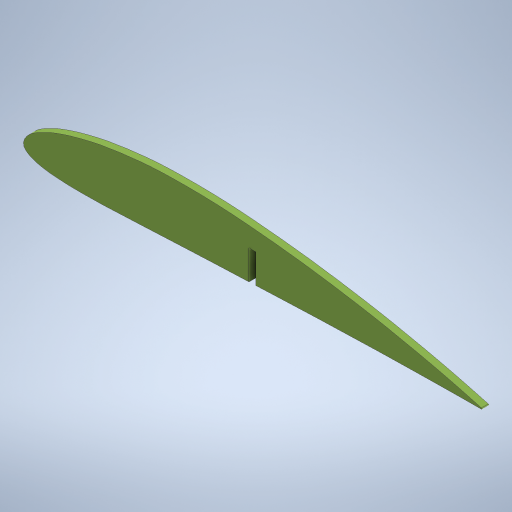
# Autodesk Inventor part: 4412_v1
Saved by Autodesk Inventor 2023 (Build 270158000, 158)
## iProperties
Created: 2023-03-24
Part Number: 4412_v1
Material: 一般
Document SubType Name: Modeling
Designer: USER
Density: 1 g/cm^3
Appearance: 預設
Author: USER
Autodesk Inventor part; units mm, degrees
ref_plane "YZ Plane" through (0, 0, 0) normal (1, 0, 0) x (0, 1, 0)
ref_plane "XZ Plane" through (0, 0, 0) normal (0, 1, 0) x (-1, 0, 0)
ref_plane "XY Plane" through (0, 0, 0) normal (0, 0, 1) x (1, 0, 0)
sketch "草圖1" plane through (0, 0, 0) normal (0, 0, 1) x (1, 0, 0)
  line L0 (0, 0) -> (200, 0)
  spline S0 degree 5 poles (200, 0.26) (199.5446, 0.3844) (198.643, 0.6302) (197.3181, 0.9903) (195.6063, 1.453) (193.5543, 2.0031) (191.5787, 2.5275) (189.6569, 3.0313) (187.7508, 3.5231) (185.8051, 4.0154) (183.7585, 4.5216) (181.5544, 5.0544) (179.1503, 5.6225) (176.5302, 6.2285) (173.7086, 6.8677) (170.7206, 7.5304) (167.6153, 8.2039) (164.4478, 8.8744) (161.2711, 9.5287) (158.1294, 10.1562) (155.049, 10.7515) (152.0374, 11.3137) (149.089, 11.8454) (146.1883, 12.3515) (143.3146, 12.838) (140.4456, 13.3106) (137.5617, 13.7738) (134.6503, 14.2291) (131.7054, 14.6761) (128.7263, 15.1128) (125.7172, 15.536) (122.6855, 15.9427) (119.6411, 16.3299) (116.5958, 16.6958) (113.5615, 17.0403) (110.5493, 17.3644) (107.5679, 17.6696) (104.622, 17.9576) (101.7109, 18.2296) (98.8272, 18.4862) (95.9547, 18.7266) (93.0695, 18.9482) (90.1456, 19.148) (87.1597, 19.3223) (84.0961, 19.4676) (80.9521, 19.5813) (77.742, 19.6616) (74.5041, 19.7086) (71.2944, 19.7241) (68.1764, 19.7106) (65.2112, 19.671) (62.448, 19.6081) (59.9142, 19.524) (57.6056, 19.4194) (55.4772, 19.2935) (53.4603, 19.1445) (51.4808, 18.9706) (49.475, 18.7707) (47.4102, 18.5458) (45.2937, 18.2988) (43.1539, 18.033) (41.0254, 17.7504) (38.934, 17.4502) (36.8779, 17.1267) (34.8276, 16.7703) (32.7467, 16.3712) (30.607, 15.9227) (28.4044, 15.4243) (26.179, 14.8861) (24.0032, 14.3258) (21.9558, 13.764) (20.1015, 13.2199) (18.469, 12.7066) (17.0265, 12.2268) (15.7021, 11.7703) (14.4082, 11.3134) (13.0653, 10.8144) (11.6221, 10.2236) (10.0713, 9.5131) (8.4648, 8.6999) (6.934, 7.8762) (5.6123, 7.1405) (4.5725, 6.5405) (3.7219, 5.9828) (2.8346, 5.2495) (1.7625, 4.1589) (0.6692, 2.7324) (-0.0769, 1.1595) (-0.1407, -0.3236) (0.5512, -1.5343) (1.6727, -2.4287) (2.8099, -3.0466) (3.7582, -3.4781) (4.6879, -3.8221) (5.8475, -4.1567) (7.301, -4.4987) (8.9432, -4.8213) (10.6131, -5.0854) (12.187, -5.2714) (13.6369, -5.3945) (14.9928, -5.4819) (16.3281, -5.5594) (17.7357, -5.6344) (19.3032, -5.7026) (21.0893, -5.7553) (23.0929, -5.7872) (25.2592, -5.798) (27.5089, -5.79) (29.7601, -5.7666) (31.9526, -5.7308) (34.0742, -5.6837) (36.1467, -5.625) (38.2074, -5.5539) (40.2921, -5.4701) (42.4166, -5.375) (44.563, -5.2721) (46.698, -5.1658) (48.7889, -5.0604) (50.8183, -4.9588) (52.8042, -4.8613) (54.8025, -4.7653) (56.8859, -4.6667) (59.127, -4.5612) (61.5817, -4.4455) (64.2685, -4.3186) (67.1689, -4.1818) (70.2406, -4.0382) (73.4254, -3.8914) (76.6596, -3.7455) (79.8838, -3.6039) (83.0524, -3.4692) (86.1437, -3.3421) (89.1553, -3.2219) (92.0991, -3.1068) (94.9966, -2.9948) (97.8733, -2.8834) (100.7544, -2.7707) (103.6595, -2.6554) (106.5987, -2.5371) (109.5748, -2.4164) (112.585, -2.2942) (115.6219, -2.1719) (118.6749, -2.0509) (121.7322, -1.9326) (124.7818, -1.8179) (127.8126, -1.7074) (130.816, -1.6015) (133.7865, -1.5002) (136.7231, -1.4033) (139.6303, -1.3107) (142.5187, -1.2221) (145.4072, -1.1373) (148.3186, -1.0562) (151.2753, -0.9786) (154.2954, -0.9047) (157.3876, -0.8343) (160.5477, -0.7676) (163.7537, -0.7048) (166.9627, -0.6461) (170.1209, -0.5918) (173.1707, -0.5421) (176.0595, -0.4974) (178.7477, -0.4575) (181.2159, -0.4226) (183.4759, -0.3922) (185.569, -0.3661) (187.5529, -0.3435) (189.4913, -0.324) (191.4427, -0.3071) (193.4484, -0.2923) (195.5324, -0.2795) (197.2722, -0.2708) (198.6195, -0.2651) (199.5367, -0.2616) (200, -0.26) knots 0 0 0 0 0 0 0.005882 0.011765 0.017647 0.023529 0.029412 0.035294 0.041176 0.047059 0.052941 0.058824 0.064706 0.070588 0.076471 0.082353 0.088235 0.094118 0.1 0.105882 0.111765 0.117647 0.123529 0.129412 0.135294 0.141176 0.147059 0.152941 0.158824 0.164706 0.170588 0.176471 0.182353 0.188235 0.194118 0.2 0.205882 0.211765 0.217647 0.223529 0.229412 0.235294 0.241176 0.247059 0.252941 0.258824 0.264706 0.270588 0.276471 0.282353 0.288235 0.294118 0.3 0.305882 0.311765 0.317647 0.323529 0.329412 0.335294 0.341176 0.347059 0.352941 0.358824 0.364706 0.370588 0.376471 0.382353 0.388235 0.394118 0.4 0.405882 0.411765 0.417647 0.423529 0.429412 0.435294 0.441176 0.447059 0.452941 0.458824 0.464706 0.470588 0.476471 0.482353 0.488235 0.494118 0.5 0.505882 0.511765 0.517647 0.523529 0.529412 0.535294 0.541176 0.547059 0.552941 0.558824 0.564706 0.570588 0.576471 0.582353 0.588235 0.594118 0.6 0.605882 0.611765 0.617647 0.623529 0.629412 0.635294 0.641176 0.647059 0.652941 0.658824 0.664706 0.670588 0.676471 0.682353 0.688235 0.694118 0.7 0.705882 0.711765 0.717647 0.723529 0.729412 0.735294 0.741176 0.747059 0.752941 0.758824 0.764706 0.770588 0.776471 0.782353 0.788235 0.794118 0.8 0.805882 0.811765 0.817647 0.823529 0.829412 0.835294 0.841176 0.847059 0.852941 0.858824 0.864706 0.870588 0.876471 0.882353 0.888235 0.894118 0.9 0.905882 0.911765 0.917647 0.923529 0.929412 0.935294 0.941176 0.947059 0.952941 0.958824 0.964706 0.970588 0.976471 0.982353 0.988235 0.994118 1 1 1 1 1 1 weights 1 1 1 1 1 1 1 1 1 1 1 1 1 1 1 1 1 1 1 1 1 1 1 1 1 1 1 1 1 1 1 1 1 1 1 1 1 1 1 1 1 1 1 1 1 1 1 1 1 1 1 1 1 1 1 1 1 1 1 1 1 1 1 1 1 1 1 1 1 1 1 1 1 1 1 1 1 1 1 1 1 1 1 1 1 1 1 1 1 1 1 1 1 1 1 1 1 1 1 1 1 1 1 1 1 1 1 1 1 1 1 1 1 1 1 1 1 1 1 1 1 1 1 1 1 1 1 1 1 1 1 1 1 1 1 1 1 1 1 1 1 1 1 1 1 1 1 1 1 1 1 1 1 1 1 1 1 1 1 1 1 1 1 1 1 1 1 1 1 1 1 1 1 1 1
  line L1 (200, 0.26) -> (199.5446, 0.3844) construction
  line L2 (199.5446, 0.3844) -> (198.643, 0.6302) construction
  line L3 (198.643, 0.6302) -> (197.3181, 0.9903) construction
  line L4 (197.3181, 0.9903) -> (195.6063, 1.453) construction
  line L5 (195.6063, 1.453) -> (193.5543, 2.0031) construction
  line L6 (193.5543, 2.0031) -> (191.5787, 2.5275) construction
  line L7 (191.5787, 2.5275) -> (189.6569, 3.0313) construction
  line L8 (189.6569, 3.0313) -> (187.7508, 3.5231) construction
  line L9 (187.7508, 3.5231) -> (185.8051, 4.0154) construction
  line L10 (185.8051, 4.0154) -> (183.7585, 4.5216) construction
  line L11 (183.7585, 4.5216) -> (181.5544, 5.0544) construction
  line L12 (181.5544, 5.0544) -> (179.1503, 5.6225) construction
  line L13 (179.1503, 5.6225) -> (176.5302, 6.2285) construction
  line L14 (176.5302, 6.2285) -> (173.7086, 6.8677) construction
  line L15 (173.7086, 6.8677) -> (170.7206, 7.5304) construction
  line L16 (170.7206, 7.5304) -> (167.6153, 8.2039) construction
  line L17 (167.6153, 8.2039) -> (164.4478, 8.8744) construction
  line L18 (164.4478, 8.8744) -> (161.2711, 9.5287) construction
  line L19 (161.2711, 9.5287) -> (158.1294, 10.1562) construction
  line L20 (158.1294, 10.1562) -> (155.049, 10.7515) construction
  line L21 (155.049, 10.7515) -> (152.0374, 11.3137) construction
  line L22 (152.0374, 11.3137) -> (149.089, 11.8454) construction
  line L23 (149.089, 11.8454) -> (146.1883, 12.3515) construction
  line L24 (146.1883, 12.3515) -> (143.3146, 12.838) construction
  line L25 (143.3146, 12.838) -> (140.4456, 13.3106) construction
  line L26 (140.4456, 13.3106) -> (137.5617, 13.7738) construction
  line L27 (137.5617, 13.7738) -> (134.6503, 14.2291) construction
  line L28 (134.6503, 14.2291) -> (131.7054, 14.6761) construction
  line L29 (131.7054, 14.6761) -> (128.7263, 15.1128) construction
  line L30 (128.7263, 15.1128) -> (125.7172, 15.536) construction
  line L31 (125.7172, 15.536) -> (122.6855, 15.9427) construction
  line L32 (122.6855, 15.9427) -> (119.6411, 16.3299) construction
  line L33 (119.6411, 16.3299) -> (116.5958, 16.6958) construction
  line L34 (116.5958, 16.6958) -> (113.5615, 17.0403) construction
  line L35 (113.5615, 17.0403) -> (110.5493, 17.3644) construction
  line L36 (110.5493, 17.3644) -> (107.5679, 17.6696) construction
  line L37 (107.5679, 17.6696) -> (104.622, 17.9576) construction
  line L38 (104.622, 17.9576) -> (101.7109, 18.2296) construction
  line L39 (101.7109, 18.2296) -> (98.8272, 18.4862) construction
  line L40 (98.8272, 18.4862) -> (95.9547, 18.7266) construction
  line L41 (95.9547, 18.7266) -> (93.0695, 18.9482) construction
  line L42 (93.0695, 18.9482) -> (90.1456, 19.148) construction
  line L43 (90.1456, 19.148) -> (87.1597, 19.3223) construction
  line L44 (87.1597, 19.3223) -> (84.0961, 19.4676) construction
  line L45 (84.0961, 19.4676) -> (80.9521, 19.5813) construction
  line L46 (80.9521, 19.5813) -> (77.742, 19.6616) construction
  line L47 (77.742, 19.6616) -> (74.5041, 19.7086) construction
  line L48 (74.5041, 19.7086) -> (71.2944, 19.7241) construction
  line L49 (71.2944, 19.7241) -> (68.1764, 19.7106) construction
  line L50 (68.1764, 19.7106) -> (65.2112, 19.671) construction
  line L51 (65.2112, 19.671) -> (62.448, 19.6081) construction
  line L52 (62.448, 19.6081) -> (59.9142, 19.524) construction
  line L53 (59.9142, 19.524) -> (57.6056, 19.4194) construction
  line L54 (57.6056, 19.4194) -> (55.4772, 19.2935) construction
  line L55 (55.4772, 19.2935) -> (53.4603, 19.1445) construction
  line L56 (53.4603, 19.1445) -> (51.4808, 18.9706) construction
  line L57 (51.4808, 18.9706) -> (49.475, 18.7707) construction
  line L58 (49.475, 18.7707) -> (47.4102, 18.5458) construction
  line L59 (47.4102, 18.5458) -> (45.2937, 18.2988) construction
  line L60 (45.2937, 18.2988) -> (43.1539, 18.033) construction
  line L61 (43.1539, 18.033) -> (41.0254, 17.7504) construction
  line L62 (41.0254, 17.7504) -> (38.934, 17.4502) construction
  line L63 (38.934, 17.4502) -> (36.8779, 17.1267) construction
  line L64 (36.8779, 17.1267) -> (34.8276, 16.7703) construction
  line L65 (34.8276, 16.7703) -> (32.7467, 16.3712) construction
  line L66 (32.7467, 16.3712) -> (30.607, 15.9227) construction
  line L67 (30.607, 15.9227) -> (28.4044, 15.4243) construction
  line L68 (28.4044, 15.4243) -> (26.179, 14.8861) construction
  line L69 (26.179, 14.8861) -> (24.0032, 14.3258) construction
  line L70 (24.0032, 14.3258) -> (21.9558, 13.764) construction
  line L71 (21.9558, 13.764) -> (20.1015, 13.2199) construction
  line L72 (20.1015, 13.2199) -> (18.469, 12.7066) construction
  line L73 (18.469, 12.7066) -> (17.0265, 12.2268) construction
  line L74 (17.0265, 12.2268) -> (15.7021, 11.7703) construction
  line L75 (15.7021, 11.7703) -> (14.4082, 11.3134) construction
  line L76 (14.4082, 11.3134) -> (13.0653, 10.8144) construction
  line L77 (13.0653, 10.8144) -> (11.6221, 10.2236) construction
  line L78 (11.6221, 10.2236) -> (10.0713, 9.5131) construction
  line L79 (10.0713, 9.5131) -> (8.4648, 8.6999) construction
  line L80 (8.4648, 8.6999) -> (6.934, 7.8762) construction
  line L81 (6.934, 7.8762) -> (5.6123, 7.1405) construction
  line L82 (5.6123, 7.1405) -> (4.5725, 6.5405) construction
  line L83 (4.5725, 6.5405) -> (3.7219, 5.9828) construction
  line L84 (3.7219, 5.9828) -> (2.8346, 5.2495) construction
  line L85 (2.8346, 5.2495) -> (1.7625, 4.1589) construction
  line L86 (1.7625, 4.1589) -> (0.6692, 2.7324) construction
  line L87 (0.6692, 2.7324) -> (-0.0769, 1.1595) construction
  line L88 (-0.0769, 1.1595) -> (-0.1407, -0.3236) construction
  line L89 (-0.1407, -0.3236) -> (0.5512, -1.5343) construction
  line L90 (0.5512, -1.5343) -> (1.6727, -2.4287) construction
  line L91 (1.6727, -2.4287) -> (2.8099, -3.0466) construction
  line L92 (2.8099, -3.0466) -> (3.7582, -3.4781) construction
  line L93 (3.7582, -3.4781) -> (4.6879, -3.8221) construction
  line L94 (4.6879, -3.8221) -> (5.8475, -4.1567) construction
  line L95 (5.8475, -4.1567) -> (7.301, -4.4987) construction
  line L96 (7.301, -4.4987) -> (8.9432, -4.8213) construction
  line L97 (8.9432, -4.8213) -> (10.6131, -5.0854) construction
  line L98 (10.6131, -5.0854) -> (12.187, -5.2714) construction
  line L99 (12.187, -5.2714) -> (13.6369, -5.3945) construction
  line L100 (13.6369, -5.3945) -> (14.9928, -5.4819) construction
  line L101 (14.9928, -5.4819) -> (16.3281, -5.5594) construction
  line L102 (16.3281, -5.5594) -> (17.7357, -5.6344) construction
  line L103 (17.7357, -5.6344) -> (19.3032, -5.7026) construction
  line L104 (19.3032, -5.7026) -> (21.0893, -5.7553) construction
  line L105 (21.0893, -5.7553) -> (23.0929, -5.7872) construction
  line L106 (23.0929, -5.7872) -> (25.2592, -5.798) construction
  line L107 (25.2592, -5.798) -> (27.5089, -5.79) construction
  line L108 (27.5089, -5.79) -> (29.7601, -5.7666) construction
  line L109 (29.7601, -5.7666) -> (31.9526, -5.7308) construction
  line L110 (31.9526, -5.7308) -> (34.0742, -5.6837) construction
  line L111 (34.0742, -5.6837) -> (36.1467, -5.625) construction
  line L112 (36.1467, -5.625) -> (38.2074, -5.5539) construction
  line L113 (38.2074, -5.5539) -> (40.2921, -5.4701) construction
  line L114 (40.2921, -5.4701) -> (42.4166, -5.375) construction
  line L115 (42.4166, -5.375) -> (44.563, -5.2721) construction
  line L116 (44.563, -5.2721) -> (46.698, -5.1658) construction
  line L117 (46.698, -5.1658) -> (48.7889, -5.0604) construction
  line L118 (48.7889, -5.0604) -> (50.8183, -4.9588) construction
  line L119 (50.8183, -4.9588) -> (52.8042, -4.8613) construction
  line L120 (52.8042, -4.8613) -> (54.8025, -4.7653) construction
  line L121 (54.8025, -4.7653) -> (56.8859, -4.6667) construction
  line L122 (56.8859, -4.6667) -> (59.127, -4.5612) construction
  line L123 (59.127, -4.5612) -> (61.5817, -4.4455) construction
  line L124 (61.5817, -4.4455) -> (64.2685, -4.3186) construction
  line L125 (64.2685, -4.3186) -> (67.1689, -4.1818) construction
  line L126 (67.1689, -4.1818) -> (70.2406, -4.0382) construction
  line L127 (70.2406, -4.0382) -> (73.4254, -3.8914) construction
  line L128 (73.4254, -3.8914) -> (76.6596, -3.7455) construction
  line L129 (76.6596, -3.7455) -> (79.8838, -3.6039) construction
  line L130 (79.8838, -3.6039) -> (83.0524, -3.4692) construction
  line L131 (83.0524, -3.4692) -> (86.1437, -3.3421) construction
  line L132 (86.1437, -3.3421) -> (89.1553, -3.2219) construction
  line L133 (89.1553, -3.2219) -> (92.0991, -3.1068) construction
  line L134 (92.0991, -3.1068) -> (94.9966, -2.9948) construction
  line L135 (94.9966, -2.9948) -> (97.8733, -2.8834) construction
  line L136 (97.8733, -2.8834) -> (100.7544, -2.7707) construction
  line L137 (100.7544, -2.7707) -> (103.6595, -2.6554) construction
  line L138 (103.6595, -2.6554) -> (106.5987, -2.5371) construction
  line L139 (106.5987, -2.5371) -> (109.5748, -2.4164) construction
  line L140 (109.5748, -2.4164) -> (112.585, -2.2942) construction
  line L141 (112.585, -2.2942) -> (115.6219, -2.1719) construction
  line L142 (115.6219, -2.1719) -> (118.6749, -2.0509) construction
  line L143 (118.6749, -2.0509) -> (121.7322, -1.9326) construction
  line L144 (121.7322, -1.9326) -> (124.7818, -1.8179) construction
  line L145 (124.7818, -1.8179) -> (127.8126, -1.7074) construction
  line L146 (127.8126, -1.7074) -> (130.816, -1.6015) construction
  line L147 (130.816, -1.6015) -> (133.7865, -1.5002) construction
  line L148 (133.7865, -1.5002) -> (136.7231, -1.4033) construction
  line L149 (136.7231, -1.4033) -> (139.6303, -1.3107) construction
  line L150 (139.6303, -1.3107) -> (142.5187, -1.2221) construction
  line L151 (142.5187, -1.2221) -> (145.4072, -1.1373) construction
  line L152 (145.4072, -1.1373) -> (148.3186, -1.0562) construction
  line L153 (148.3186, -1.0562) -> (151.2753, -0.9786) construction
  line L154 (151.2753, -0.9786) -> (154.2954, -0.9047) construction
  line L155 (154.2954, -0.9047) -> (157.3876, -0.8343) construction
  line L156 (157.3876, -0.8343) -> (160.5477, -0.7676) construction
  line L157 (160.5477, -0.7676) -> (163.7537, -0.7048) construction
  line L158 (163.7537, -0.7048) -> (166.9627, -0.6461) construction
  line L159 (166.9627, -0.6461) -> (170.1209, -0.5918) construction
  line L160 (170.1209, -0.5918) -> (173.1707, -0.5421) construction
  line L161 (173.1707, -0.5421) -> (176.0595, -0.4974) construction
  line L162 (176.0595, -0.4974) -> (178.7477, -0.4575) construction
  line L163 (178.7477, -0.4575) -> (181.2159, -0.4226) construction
  line L164 (181.2159, -0.4226) -> (183.4759, -0.3922) construction
  line L165 (183.4759, -0.3922) -> (185.569, -0.3661) construction
  line L166 (185.569, -0.3661) -> (187.5529, -0.3435) construction
  line L167 (187.5529, -0.3435) -> (189.4913, -0.324) construction
  line L168 (189.4913, -0.324) -> (191.4427, -0.3071) construction
  line L169 (191.4427, -0.3071) -> (193.4484, -0.2923) construction
  line L170 (193.4484, -0.2923) -> (195.5324, -0.2795) construction
  line L171 (195.5324, -0.2795) -> (197.2722, -0.2708) construction
  line L172 (197.2722, -0.2708) -> (198.6195, -0.2651) construction
  line L173 (198.6195, -0.2651) -> (199.5367, -0.2616) construction
  line L174 (199.5367, -0.2616) -> (200, -0.26) construction
  spline S1 degree 5 poles (200, 0.26) (200.0553, 0.2263) (200.15, 0.1598) (200.2445, 0.0626) (200.2695, -0.0428) (200.1977, -0.1428) (200.0974, -0.2107) (200.0224, -0.2492) (200, -0.26) knots 0 0 0 0 0 0 0.294912 0.589823 0.884735 1 1 1 1 1 1 weights 1 1 1 1 1 1 1 1 1
  line L175 (200, 0.26) -> (200.0553, 0.2263) construction
  line L176 (200.0553, 0.2263) -> (200.15, 0.1598) construction
  line L177 (200.15, 0.1598) -> (200.2445, 0.0626) construction
  line L178 (200.2445, 0.0626) -> (200.2695, -0.0428) construction
  line L179 (200.2695, -0.0428) -> (200.1977, -0.1428) construction
  line L180 (200.1977, -0.1428) -> (200.0974, -0.2107) construction
  line L181 (200.0974, -0.2107) -> (200.0224, -0.2492) construction
  line L182 (200.0224, -0.2492) -> (200, -0.26) construction
  point P0 (200.0013, -0.2594)
  constraints: 2 end point, 5 other
extrude "擠出1" add sketch "草圖1" along normal blind 3
sketch "草圖2" plane through (0, 0, 3) normal (0, 0, 1) x (1, 0, 0)
  line L0 (98.5, 10) -> (101.5, 10)
  line L1 (101.5, 10) -> (101.5, -5)
  line L2 (101.5, -5) -> (98.5, -5)
  line L3 (98.5, -5) -> (98.5, 10)
  line L4 (-40.2228, 0) -> (240.3516, 0) projected
  point P0 (0, 0)
  point P1 (100, 10)
  dimension "d2" = 3
  dimension "d3" = 100
  dimension "d4" = 10
  dimension "d5" = 15
  constraints: 8 end point, 2 parallel, 1 horizontal, 1 midpoint, 1 perpendicular
  measures "d2" distance of L1.end L2.end
  measures "d3" horizontal distance of point (0, 0) point (100, 10)
  measures "d4" distance from line of L4 point (100, 10)
  measures "d5" distance between parallel lines of L0 L2
extrude "擠出2" cut sketch "草圖2" against normal through all
